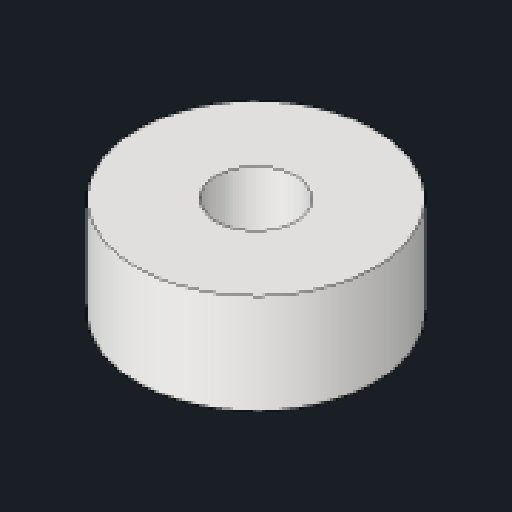
# Autodesk Inventor part: 2x6x2.5mm Bearing
Saved by Autodesk Inventor 2023.2 (Build 272271030, 271C)
## iProperties
Created: 2024-02-20
Part Number: 2x6x2.5mm Bearing
Material: Generic
Document SubType Name: Modeling
Designer: robpl
Density: 1 g/cm^3
Appearance: Default
Author: robpl
Autodesk Inventor part; units mm, degrees
ref_plane "YZ Plane" through (0, 0, 0) normal (1, 0, 0) x (0, 1, 0)
ref_plane "XZ Plane" through (0, 0, 0) normal (0, 1, 0) x (-1, 0, 0)
ref_plane "XY Plane" through (0, 0, 0) normal (0, 0, 1) x (1, 0, 0)
sketch "Sketch1" plane through (0, 0, 0) normal (0, 0, 1) x (1, 0, 0)
  line L0 (3, 1.25) -> (1, 1.25)
  line L1 (1, 1.25) -> (1, -1.25)
  line L2 (1, -1.25) -> (3, -1.25)
  line L3 (3, -1.25) -> (3, 1.25)
  line L4 (0, 0) -> (0, -1.4359)
  point P0 (3, 0)
  dimension "d0" = 3
  dimension "d1" = 1
  dimension "d2" = 2.5
  constraints: 10 end point, 2 parallel, 1 horizontal, 1 horizontal alignment, 1 midpoint, 1 perpendicular, 1 vertical
  measures "d0" distance from line of L4.start L3
  measures "d1" distance from line of L4.start L1
  measures "d2" distance of L2.end L0.start
revolve "Revolution1" add sketch "Sketch1" angle 360 about axis through (0, 0, 0) along (0, -1, 0)
body "Solid1"
